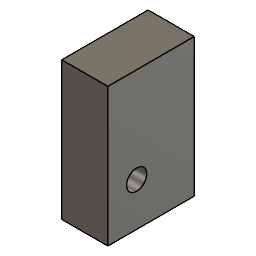
replay (Autodesk Fusion 360 design; units mm, degrees)
Autodesk Fusion 360 part; units mm, degrees
ref_plane "工作平面1" through (-2, 0, 0) normal (1, 0, 0) x (0, 1, 0)
sketch "草图1" plane through (-2, 0, 0) normal (1, 0, 0) x (0, 0, -1)
  line L0 (-3, 43) -> (-33, 43)
  line L1 (-33, 43) -> (-33, -5)
  line L2 (-33, -5) -> (-3, -5)
  line L3 (-3, -5) -> (-3, 43)
extrude "拉伸1" add sketch "草图1" along normal blind 16
sketch "草图2" plane through (14, 0, 0) normal (1, 0, 0) x (0, 0, -1)
  line L0 (-3, -5) -> (-3, 43)
  line L1 (-3, 43) -> (-33, 43)
  line L2 (-33, 43) -> (-33, -5)
  line L3 (-33, -5) -> (-3, -5)
  circle A0 centre (-23, 10) radius 3.5
extrude "拉伸2" cut sketch "草图2" against normal through all contours A0
